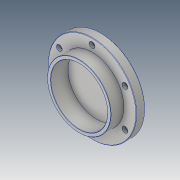
# Autodesk Inventor part: 200-10-ROCKER-BEARING-02
Saved by Autodesk Inventor 2018.1 (Build 221171000, 171)
## iProperties
Created: 2017-10-26
Part Number: 200-10-ROCKER-BEARING-02
Material: Aluminium 6061
Document SubType Name: Modeling
Designer: marti
Density: 2.7 g/cm^3
Appearance: Aluminium - flach
Author: marti
Autodesk Inventor part; units mm, degrees
ref_plane "YZ Plane" through (0, 0, 0) normal (1, 0, 0) x (0, 1, 0)
ref_plane "XZ Plane" through (0, 0, 0) normal (0, 1, 0) x (-1, 0, 0)
ref_plane "XY Plane" through (0, 0, 0) normal (0, 0, 1) x (1, 0, 0)
derived "200-10-ROCKER-BEARING-01.ipt"
sketch "Skizze_Lagersitz" plane through (0, 0, 0) normal (1, 0, 0) x (0, 1, 0)
  line L0 (-12.5, 36) -> (32.5, 36)
  line L1 (-12.5, -36) -> (-12.5, 36)
  line L2 (-17.5, 32.25) -> (-12.5, 32.25)
  line L3 (-17.5, -32.25) -> (-17.5, 32.25)
  line L4 (-32.5, 18) -> (-17.5, 18)
  line L5 (-32.5, -18) -> (-17.5, -18)
  line L6 (-17.5, -32.25) -> (-12.5, -32.25)
  line L7 (-12.5, -36) -> (32.5, -36)
  line L8 (32.5, 36) -> (32.5, -36)
  line L9 (32.5, 50) -> (32.5, -50)
  line L10 (30, -50) -> (30, 0)
  line L11 (-32.5, -18) -> (-32.5, 18)
  line L12 (-32.5, 50) -> (-32.5, -50)
  line L13 (-32.5, -50) -> (-32.5, 50)
  line L14 (-12.5, -36) -> (-12.5, 36)
  point P0 (0, 0)
  point P1 (30, 86)
  point P2 (30, 14)
  point P3 (-30, 32)
  point P4 (-30, 68)
sketch "Skizze4" plane through (0, 0, 0) normal (1, 0, 0) x (0, 1, 0)
  line L0 (-12.5, -36) -> (-12.5, 36) construction
  line L1 (32.5, 36) -> (32.5, -36) construction
  line L2 (32.5, 50) -> (42.5, 50)
  line L3 (32.5, 36) -> (17.7, 36)
  line L4 (17.7, 36) -> (17.7, 32.25)
  line L5 (17.7, 32.25) -> (37.5, 32.25)
  line L6 (-17.5, 32.25) -> (-12.5, 32.25) construction
  line L7 (32.5, 36) -> (32.5, 50)
  line L8 (32.5, 36) -> (32.5, -36) construction
  line L9 (42.5, 50) -> (42.5, 0)
  line L10 (42.5, 0) -> (37.5, 0)
  line L11 (37.5, 0) -> (37.5, 32.25)
  line L12 (-51, 0) -> (61, 0) construction
  point P0 (0, 0)
  point P1 (-15, 32.25)
  dimension "d34" = 30.2
  dimension "d73" = 10
  dimension "d74" = 5
  constraints: 18 end point, 4 perpendicular, 2 horizontal, 2 horizontal alignment, 2 point on line, 1 midpoint, 1 vertical
  measures "d34" distance between parallel lines of L4 L0
  measures "d73" distance between parallel lines of L9 L7
  measures "d74" distance between parallel lines of L9 L11
revolve "Grundkoerper" add sketch "Skizze4" angle 360 about axis through (0, 0, 0) along (0, 1, 0)
sketch "Skizze6" plane through (0, 42.5, 0) normal (0, 1, 0) x (1, 0, 0)
  circle A0 centre (0, 0) radius 36 construction
  circle A1 centre (0, 0) radius 50 construction
  circle A2 centre (0, 0) radius 43 construction
  line L0 (0, 77.2) -> (0, -113.2) construction
  line L1 (70, 0) -> (-70, 0) construction
  point P0 (0, -43)
  point P1 (37.2391, -21.5)
  point P2 (37.2391, 21.5)
  point P3 (0, 43)
  point P4 (-37.2391, 21.5)
  point P5 (-37.2391, -21.5)
  dimension "d59" = 86
  dimension "d57" = 72
  dimension "d58" = 100
  dimension "d62" = 360
  constraints: 1 coincident, 1 point on line, 1 vertical alignment, 9 other
  measures "d57" diameter of A0
  measures "d58" diameter of A1
hole "M6_Boh" at (0, 42.5, 43) at (37.2391, 42.5, 21.5) at (37.2391, 42.5, -21.5) at (0, 42.5, -43) at (-37.2391, 42.5, -21.5) at (-37.2391, 42.5, 21.5) direction (0, -1, 0) diameter 6.6 end through all counterbore diameter 11 counterbore depth 6.4
chamfer "Fase_Passung" distance 0.3 angle 45 2 edges at (0, 17.7, -32.25) (0, 17.7, -36)
chamfer "Fase_Allgemein" distance 0.5 angle 45 2 edges at (0, 32.5, -50) (0, 42.5, -50)
equation "\"d59\" = 0.5 * d58 + 0.5 * d57"
